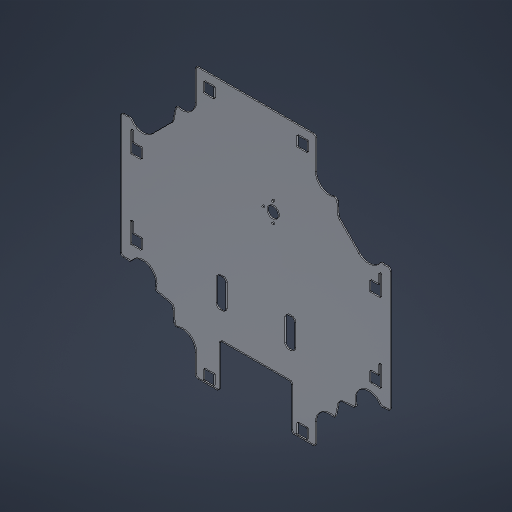
# Autodesk Inventor part: PLATE,BELLYPAN
Saved by Autodesk Inventor 2026 (Build 300175000, 175)
## iProperties
Created: 2026-01-19
Part Number: PLATE,BELLYPAN
Material: Polycarbonate, Clear
Document SubType Name: Sheet Metal
Designer: Jthib
Mass: 1216.4 g
Surface Area: 6786.66 cm^2
Volume: 1013.67 cm^3
Density: 1.2 g/cm^3
Sheet Metal Rule: Default
Appearance: Polycarbonate - Clear
Author: Jthib
Autodesk Inventor part; units mm, degrees
ref_plane "YZ Plane" through (0, 0, 0) normal (1, 0, 0) x (0, 1, 0)
ref_plane "XZ Plane" through (0, 0, 0) normal (0, 1, 0) x (-1, 0, 0)
ref_plane "XY Plane" through (0, 0, 0) normal (0, 0, 1) x (1, 0, 0)
sketch "Sketch1" plane through (0, 0, 0) normal (0, 0, 1) x (1, 0, 0)
  line L0 (-298.45, -349.25) -> (298.45, -349.25)
  line L1 (349.25, -298.45) -> (349.25, 298.45)
  line L2 (298.45, 349.25) -> (-298.45, 349.25)
  line L3 (-349.25, 298.45) -> (-349.25, -298.45)
  line L4 (-349.25, -349.25) -> (349.25, 349.25) construction
  line L5 (349.25, -349.25) -> (-349.25, 349.25) construction
  arc A0 (349.25, 298.45) -> (298.45, 349.25) centre (298.45, 298.45) ccw
  arc A1 (-298.45, 349.25) -> (-349.25, 298.45) centre (-298.45, 298.45) ccw
  arc A2 (-349.25, -298.45) -> (-298.45, -349.25) centre (-298.45, -298.45) ccw
  arc A3 (298.45, -349.25) -> (349.25, -298.45) centre (298.45, -298.45) ccw
  point P0 (0, 0)
  dimension "d0" = 698.5
  dimension "d4" = 50.8
  measures "d0" distance of L4.end L5.end
  measures "d4" radius of A0
extrude "Plate1" add sketch "Sketch1" along normal blind 3.048
sketch "Sketch2" plane through (0, 0, 0) normal (0, 0, -1) x (-1, 0, 0)
  line L0 (-188.9125, -349.25) -> (-336.55, -349.25)
  line L1 (-179.3875, -333.375) -> (-179.3875, -339.725) construction
  arc A0 (-179.3875, -333.375) -> (-188.9125, -323.85) centre (-188.9125, -333.375) ccw construction
  line L2 (-190.5, -323.85) -> (-188.9125, -323.85) construction
  arc A1 (-221.4273, -289.3223) -> (-190.5, -323.85) centre (-190.5, -292.735) ccw construction
  arc A2 (-349.25, -336.55) -> (-336.55, -349.25) centre (-336.55, -336.55) ccw
  line L3 (-349.25, -336.55) -> (-349.25, -188.9125)
  line L4 (-339.725, -179.3875) -> (-333.375, -179.3875) construction
  arc A3 (-323.85, -188.9125) -> (-333.375, -179.3875) centre (-333.375, -188.9125) ccw construction
  line L5 (-323.85, -188.9125) -> (-323.85, -190.5) construction
  arc A4 (-323.85, -190.5) -> (-289.3223, -221.4273) centre (-292.735, -190.5) ccw construction
  arc A5 (-213.9609, -272.2965) -> (-221.4273, -289.3223) centre (-190.5, -292.735) ccw construction
  arc A6 (-213.9609, -272.2965) -> (-211.7954, -264.058) centre (-221.2002, -265.9898) ccw construction
  line L6 (-220.0695, -223.7764) -> (-211.7954, -264.058) construction
  arc A7 (-220.0695, -223.7764) -> (-224.3016, -219.9918) centre (-224.7346, -224.7346) ccw construction
  line L7 (-270.7455, -215.751) -> (-224.3016, -219.9918) construction
  arc A8 (-270.7455, -215.751) -> (-276.598, -217.1034) centre (-271.6186, -225.3124) ccw construction
  arc A9 (-289.3223, -221.4273) -> (-276.598, -217.1034) centre (-292.735, -190.5) ccw construction
  line L8 (-179.3875, -339.725) -> (-179.3875, -349.25) construction
  line L9 (-173.0375, -349.25) -> (-188.9125, -349.25)
  line L10 (-349.25, -188.9125) -> (-349.25, -173.0375)
  line L11 (-349.25, -179.3875) -> (-339.725, -179.3875) construction
  line L12 (-333.375, -173.0375) -> (-339.9898, -173.0375)
  line L13 (-339.9898, -173.0375) -> (-349.25, -173.0375)
  line L14 (-173.0375, -349.25) -> (-173.0375, -339.725)
  line L15 (-173.0375, -339.725) -> (-173.0375, -333.375)
  arc A10 (-173.0375, -333.375) -> (-188.9125, -317.5) centre (-188.9125, -333.375) ccw
  line L16 (-188.9125, -317.5) -> (-190.5, -317.5)
  arc A11 (-215.1156, -290.0188) -> (-190.5, -317.5) centre (-190.5, -292.735) ccw
  arc A12 (-209.1729, -276.4676) -> (-215.1156, -290.0188) centre (-190.5, -292.735) ccw
  arc A13 (-209.1729, -276.4676) -> (-205.5752, -262.7803) centre (-221.2002, -265.9898) ccw
  line L17 (-205.5752, -262.7803) -> (-213.8494, -222.4987)
  arc A14 (-213.8494, -222.4987) -> (-223.7241, -213.6682) centre (-224.7346, -224.7346) ccw
  line L18 (-223.7241, -213.6682) -> (-270.1681, -209.4273)
  arc A15 (-270.1681, -209.4273) -> (-279.8913, -211.6741) centre (-271.6186, -225.3124) ccw
  arc A16 (-290.0188, -215.1156) -> (-279.8913, -211.6741) centre (-292.735, -190.5) ccw
  arc A17 (-317.5, -190.5) -> (-290.0188, -215.1156) centre (-292.735, -190.5) ccw
  line L19 (-317.5, -190.5) -> (-317.5, -188.9125)
  arc A18 (-317.5, -188.9125) -> (-333.375, -173.0375) centre (-333.375, -188.9125) ccw
  line L20 (298.45, -349.25) -> (-298.45, -349.25) construction
  circle A19 centre (-190.5, -292.735) radius 34.925
  circle A20 centre (-292.735, -190.5) radius 34.925
  point P0 (0, 0)
  point P1 (-263.7686, -210.0117)
  point P2 (-324.4183, -175.8055)
  point P3 (-175.8055, -324.4183)
  point P4 (-205.8647, -261.3713)
  dimension "d9" = 6.35
  dimension "d19" = 69.85
  constraints: 40 end point, 38 point on circle, 21 centre point, 5 vertical, 3 horizontal, 3 perpendicular, 2 coincident, 2 collinear, 2 point on line, 1 equal radius, 1 tangent, 55 other
  measures "d9" distance between parallel lines of L17 L6
  measures "d19" diameter of A19
extrude "Cut1" cut sketch "Sketch2" against normal blind 3.048
fillet "Corner Round2" radius 6.35 4 edges at (205.8647, -261.3713, 1.524) (175.8055, -324.4183, 1.524) (263.7686, -210.0117, 1.524) (324.4183, -175.8055, 1.524)
pattern_circular "Circular Pattern1" count 4 over 360 about axis through (0, 0, -10) along (0, 0, 1) of "Cut1", "Corner Round2"
sketch "Sketch3" plane through (0, 0, 0) normal (0, 0, -1) x (-1, 0, 0)
  line L0 (-173.0375, 349.25) -> (173.0375, 349.25) projected
  line L1 (-349.25, -173.0375) -> (-349.25, 173.0375) projected
  point P0 (0, 0)
  point P1 (-44.45, 120.65)
  point P2 (-166.6875, 349.25)
  point P3 (166.6875, 349.25)
  point P4 (-349.25, -166.6875)
  point P5 (-349.25, 166.6875)
  dimension "d10" = 228.6
  dimension "d11" = 304.8
  measures "d10" distance from line of L0 point (-44.45, 120.65)
  measures "d11" distance from line of L1 point (-44.45, 120.65)
hole "Hole1" at (44.45, 120.65, 0) direction (0, 0, 1) diameter 28.575 end through all
sketch "Sketch4" plane through (0, 0, 0) normal (0, 0, -1) x (-1, 0, 0)
  line L0 (173.0375, -349.25) -> (-173.0375, -349.25) construction
  line L1 (93.6625, -349.25) -> (-93.6625, -349.25)
  line L2 (-93.6625, -349.25) -> (-93.6625, -234.95)
  line L3 (-93.6625, -234.95) -> (93.6625, -234.95)
  line L4 (93.6625, -234.95) -> (93.6625, -349.25)
  line L5 (0, -488.95) -> (0, 488.95) construction
  point P0 (0, 0)
  point P1 (166.6875, -349.25)
  point P2 (-166.6875, -349.25)
  dimension "d21" = 187.325
  dimension "d22" = 114.3
  constraints: 8 end point, 2 parallel, 1 horizontal, 1 perpendicular, 1 point on line, 1 other
  measures "d21" distance of L1.start L1.end
  measures "d22" distance of L1.end L2.end
extrude "Cut2" cut sketch "Sketch4" against normal blind 3.048
sketch "Sketch5" plane through (0, 0, 0) normal (0, 0, -1) x (-1, 0, 0)
  line L0 (0, -488.95) -> (0, 488.95) construction
  circle A0 centre (-44.3766, 95.1768) radius 2.0193 construction
  circle A1 centre (-19.05, 120.65) radius 2.0193 construction
  circle A2 centre (-44.5232, 145.9766) radius 2.0193 construction
  point P0 (0, 0)
  constraints: 3 centre point, 6 other
hole "Hole2" at (44.3766, 95.1768, 0) at (19.05, 120.65, 0) at (44.5232, 145.9766, 0) direction (0, 0, 1) diameter 5.1054 end through all start extended yes clearance for "Flat Head Machine Screw (82)" size "#10" standard "Ansi Unified Screw Threads"
sketch "Sketch6" plane through (0, 0, 0) normal (0, 0, -1) x (-1, 0, 0)
  circle A0 centre (-44.5232, 145.9766) radius 2.5527 construction
  circle A1 centre (-19.05, 120.65) radius 2.5527 construction
  circle A2 centre (-44.3766, 95.1768) radius 2.5527 construction
  line L0 (93.6625, -234.95) -> (93.6625, -349.25) construction
  line L1 (173.0375, -349.25) -> (93.6625, -349.25) projected
  line L2 (173.0375, -349.25) -> (173.0375, -333.375) projected
  arc A3 (173.6888, -328.8745) -> (173.0375, -333.375) centre (188.9125, -333.375) ccw projected
  arc A4 (173.6888, -328.8745) -> (171.1225, -321.7913) centre (167.5993, -327.0743) ccw projected
  arc A5 (202.3754, -259.891) -> (171.1225, -321.7913) centre (190.5, -292.735) ccw projected
  arc A6 (202.3754, -259.891) -> (210.8583, -254.4968) centre (204.5346, -253.9193) ccw construction
  line L3 (210.8583, -254.4968) -> (213.6682, -223.7241) construction
  arc A7 (222.4987, -213.8494) -> (213.6682, -223.7241) centre (224.7346, -224.7346) ccw construction
  line L4 (222.4987, -213.8494) -> (254.1305, -207.352) construction
  arc A8 (254.1305, -207.352) -> (258.9885, -199.4962) centre (252.8528, -201.1318) ccw construction
  arc A9 (321.7913, -171.1225) -> (258.9885, -199.4962) centre (292.735, -190.5) ccw construction
  arc A10 (321.7913, -171.1225) -> (328.8745, -173.6888) centre (327.0743, -167.5993) ccw construction
  arc A11 (333.375, -173.0375) -> (328.8745, -173.6888) centre (333.375, -188.9125) ccw construction
  line L5 (333.375, -173.0375) -> (349.25, -173.0375) construction
  line L6 (349.25, 173.0375) -> (349.25, -173.0375) construction
  line L7 (349.25, 173.0375) -> (333.375, 173.0375) construction
  arc A12 (328.8745, 173.6888) -> (333.375, 173.0375) centre (333.375, 188.9125) ccw construction
  arc A13 (328.8745, 173.6888) -> (321.7913, 171.1225) centre (327.0743, 167.5993) ccw construction
  arc A14 (259.891, 202.3754) -> (321.7913, 171.1225) centre (292.735, 190.5) ccw projected
  arc A15 (259.891, 202.3754) -> (254.4968, 210.8583) centre (253.9193, 204.5346) ccw projected
  line L8 (254.4968, 210.8583) -> (223.7241, 213.6682) projected
  arc A16 (213.8494, 222.4987) -> (223.7241, 213.6682) centre (224.7346, 224.7346) ccw projected
  line L9 (213.8494, 222.4987) -> (207.352, 254.1305) construction
  arc A17 (207.352, 254.1305) -> (199.4962, 258.9885) centre (201.1318, 252.8528) ccw construction
  arc A18 (171.1225, 321.7913) -> (199.4962, 258.9885) centre (190.5, 292.735) ccw projected
  arc A19 (171.1225, 321.7913) -> (173.6888, 328.8745) centre (167.5993, 327.0743) ccw projected
  arc A20 (173.0375, 333.375) -> (173.6888, 328.8745) centre (188.9125, 333.375) ccw projected
  line L10 (173.0375, 333.375) -> (173.0375, 349.25) projected
  line L11 (-173.0375, 349.25) -> (173.0375, 349.25) projected
  line L12 (-173.0375, 349.25) -> (-173.0375, 333.375) projected
  arc A21 (-173.6888, 328.8745) -> (-173.0375, 333.375) centre (-188.9125, 333.375) ccw projected
  arc A22 (-173.6888, 328.8745) -> (-171.1225, 321.7913) centre (-167.5993, 327.0743) ccw projected
  arc A23 (-202.3754, 259.891) -> (-171.1225, 321.7913) centre (-190.5, 292.735) ccw projected
  arc A24 (-202.3754, 259.891) -> (-210.8583, 254.4968) centre (-204.5346, 253.9193) ccw construction
  line L13 (-210.8583, 254.4968) -> (-213.6682, 223.7241) construction
  arc A25 (-222.4987, 213.8494) -> (-213.6682, 223.7241) centre (-224.7346, 224.7346) ccw projected
  line L14 (-222.4987, 213.8494) -> (-254.1305, 207.352) projected
  arc A26 (-254.1305, 207.352) -> (-258.9885, 199.4962) centre (-252.8528, 201.1318) ccw projected
  arc A27 (-321.7913, 171.1225) -> (-258.9885, 199.4962) centre (-292.735, 190.5) ccw projected
  arc A28 (-321.7913, 171.1225) -> (-328.8745, 173.6888) centre (-327.0743, 167.5993) ccw construction
  arc A29 (-333.375, 173.0375) -> (-328.8745, 173.6888) centre (-333.375, 188.9125) ccw construction
  line L15 (-333.375, 173.0375) -> (-349.25, 173.0375) construction
  line L16 (-349.25, -173.0375) -> (-349.25, 173.0375) construction
  line L17 (-349.25, -173.0375) -> (-333.375, -173.0375) construction
  arc A30 (-328.8745, -173.6888) -> (-333.375, -173.0375) centre (-333.375, -188.9125) ccw construction
  arc A31 (-328.8745, -173.6888) -> (-321.7913, -171.1225) centre (-327.0743, -167.5993) ccw construction
  arc A32 (-259.891, -202.3754) -> (-321.7913, -171.1225) centre (-292.735, -190.5) ccw construction
  arc A33 (-259.891, -202.3754) -> (-254.4968, -210.8583) centre (-253.9193, -204.5346) ccw construction
  line L18 (-254.4968, -210.8583) -> (-223.7241, -213.6682) construction
  arc A34 (-213.8494, -222.4987) -> (-223.7241, -213.6682) centre (-224.7346, -224.7346) ccw construction
  line L19 (-213.8494, -222.4987) -> (-207.352, -254.1305) construction
  arc A35 (-207.352, -254.1305) -> (-199.4962, -258.9885) centre (-201.1318, -252.8528) ccw construction
  arc A36 (-171.1225, -321.7913) -> (-199.4962, -258.9885) centre (-190.5, -292.735) ccw projected
  arc A37 (-171.1225, -321.7913) -> (-173.6888, -328.8745) centre (-167.5993, -327.0743) ccw projected
  arc A38 (-173.0375, -333.375) -> (-173.6888, -328.8745) centre (-188.9125, -333.375) ccw projected
  line L20 (-173.0375, -333.375) -> (-173.0375, -349.25) projected
  line L21 (-93.6625, -349.25) -> (-173.0375, -349.25) projected
  line L22 (-93.6625, -349.25) -> (-93.6625, -234.95) construction
  line L23 (-93.6625, -234.95) -> (93.6625, -234.95) construction
  circle A39 centre (-44.45, 120.65) radius 14.2875 construction
  line L24 (155.575, -292.735) -> (155.575, -349.25)
  line L25 (-155.575, -349.25) -> (-155.575, -292.735)
  line L26 (-93.6625, -349.25) -> (-173.0375, -349.25) projected
  line L27 (155.575, 292.735) -> (155.575, 349.25)
  line L28 (-155.575, 292.735) -> (-155.575, 349.25)
  line L29 (268.061, 165.7826) -> (216.8838, 216.87)
  line L30 (-216.8838, 216.87) -> (-268.061, 165.7826)
  point P0 (0, 0)
  constraints: 12 end point, 8 point on circle, 8 tangent, 4 perpendicular, 4 point on line
extrude "Cut3" cut sketch "Sketch6" against normal blind 3.048
move faces "Move1" translate (0, -25.4, 0) faces at (-176.1603, 39.0974, 0) (-233.9429, 199.8409, 1.016) (-216.3906, 217.3953, 2.032) (-209.5178, 243.5865, 2.032) (-158.0862, 279.7312, 2.032) (-155.575, 330.4117, 1.016) (-285.9517, 156.2401, 2.032) (-325.3406, 173.7081, 2.032) (-329.3629, 173.5529, 1.016) (-338.6667, 173.0375, 1.016) (-206.407, 256.3877, 1.016) (251.0019, 182.8117, 1.016) (306.1288, 158.2453, 2.032) (213.7791, 222.8732, 2.032) (212.7315, 233.9817, 1.016) (210.3944, 256.3658, 1.016) (171.4652, 263.4531, 2.032) (155.575, 311.5733, 1.016) (324.4927, 173.4009, 2.032) (330.8507, 173.2395, 2.032) (343.9583, 173.0375, 1.016)
sketch "Sketch7" plane through (155.575, 349.25, 0) normal (0, 0, -1) x (-1, 0, 0)
  line L0 (155.575, -838.2) -> (155.575, 139.7) construction
  line L1 (0, 0) -> (311.15, 0) construction
  line L2 (479.425, -432.1175) -> (479.425, -482.2825)
  line L3 (477.8375, -483.87) -> (453.0725, -483.87)
  line L4 (451.485, -482.2825) -> (451.485, -458.7875)
  line L5 (453.0725, -457.2) -> (473.075, -457.2)
  line L6 (474.6625, -455.6125) -> (474.6625, -432.1175)
  line L7 (476.25, -430.53) -> (477.8375, -430.53)
  line L8 (504.825, -201.6125) -> (504.825, -522.2875) construction
  arc A0 (479.425, -432.1175) -> (477.8375, -430.53) centre (477.8375, -432.1175) ccw
  arc A1 (476.25, -430.53) -> (474.6625, -432.1175) centre (476.25, -432.1175) ccw
  arc A2 (473.075, -457.2) -> (474.6625, -455.6125) centre (473.075, -455.6125) ccw
  arc A3 (453.0725, -457.2) -> (451.485, -458.7875) centre (453.0725, -458.7875) ccw
  arc A4 (451.485, -482.2825) -> (453.0725, -483.87) centre (453.0725, -482.2825) ccw
  arc A5 (477.8375, -483.87) -> (479.425, -482.2825) centre (477.8375, -482.2825) ccw
  arc A6 (273.7282, -685.927) -> (278.7218, -685.927) centre (276.225, -685.8) ccw construction
  line L9 (262.89, -668.02) -> (289.56, -668.02)
  line L10 (289.56, -668.02) -> (289.56, -694.69)
  line L11 (289.56, -694.69) -> (262.89, -694.69)
  line L12 (262.89, -694.69) -> (262.89, -668.02)
  line L13 (262.89, -668.02) -> (289.56, -694.69) construction
  line L14 (289.56, -668.02) -> (262.89, -694.69) construction
  line L15 (311.15, -698.5) -> (249.2375, -698.5) construction
  point P0 (155.575, -349.25)
  point P1 (479.425, -430.53)
  point P2 (479.425, -483.87)
  point P3 (451.485, -483.87)
  point P4 (474.6625, -457.2)
  point P5 (474.6625, -430.53)
  point P6 (276.225, -681.355)
  dimension "d44" = 4.7625
  dimension "d45" = 53.34
  dimension "d46" = 26.67
  dimension "d47" = 25.4
  dimension "d48" = 27.94
  dimension "d49" = 1.5875
  dimension "d55" = 26.67
  dimension "d56" = 26.67
  dimension "d57" = 3.81
  dimension "d64" = 134.62
  constraints: 24 end point, 14 point on circle, 12 tangent, 10 point on line, 7 centre point, 6 perpendicular, 5 equal radius, 2 midpoint, 2 parallel, 1 horizontal, 1 vertical, 1 vertical alignment, 4 other
  measures "d44" distance of point (474.663, -430.53) point (479.425, -430.53)
  measures "d45" distance of point (479.425, -430.53) point (479.425, -483.87)
  measures "d46" distance of point (474.663, -457.2) point (474.663, -430.53)
  measures "d47" distance between parallel lines of L8 L2
  measures "d48" distance of point (479.425, -483.87) point (451.485, -483.87)
  measures "d49" radius of A0
  measures "d55" distance of L10.end L11.end
  measures "d56" distance of L10.end L9.end
  measures "d57" distance between parallel lines of L15 L11
  measures "d64" distance from line of point (155.575, -349.25) L3
extrude "Cut4" cut sketch "Sketch7" against normal blind 3.048 contours L2 A5 L3 A4 L4 A3 L5 A2 L6 A1 L7 A0
pattern_linear "Rectangular Pattern1" count 2 spacing 203.2 along (0, 1, 0) of "Cut4"
extrude "Cut5" cut sketch "Sketch7" against normal blind 3.048 contours L9 L10 L11 L12
pattern_linear "Rectangular Pattern2" count 2 spacing 644.525 along (0, 1, 0) of "Cut5"
sketch "Sketch8" plane through (155.575, 349.25, 0) normal (0, 0, -1) x (-1, 0, 0)
  line L0 (257.175, -514.35) -> (231.775, -514.35)
  line L1 (231.775, -514.35) -> (231.775, -438.15)
  line L2 (231.775, -438.15) -> (257.175, -438.15)
  line L3 (257.175, -438.15) -> (257.175, -514.35)
  line L4 (257.175, -514.35) -> (231.775, -438.15) construction
  line L5 (231.775, -514.35) -> (257.175, -438.15) construction
  line L6 (155.575, -838.2) -> (155.575, 139.7) construction
  line L7 (644.525, -349.25) -> (-333.375, -349.25) construction
  point P0 (155.575, -349.25)
  point P1 (244.475, -476.25)
  dimension "d66" = 76.2
  dimension "d67" = 25.4
  dimension "d68" = 76.2
  dimension "d69" = 127
  constraints: 12 end point, 2 midpoint, 2 parallel, 1 horizontal, 1 perpendicular
  measures "d66" distance of L0.end L1.end
  measures "d67" distance of L0.start L0.end
  measures "d68" distance between parallel lines of L6 L1
  measures "d69" distance from line of L7 point (244.475, -476.25)
extrude "Cut6" cut sketch "Sketch8" against normal blind 3.048
mirror "Mirror1" about plane through (0, 0, 0) normal (1, 0, 0) of "Cut4", "Rectangular Pattern1", "Cut5", "Rectangular Pattern2", "Cut6"
fillet "Corner Round3" radius 6.35 12 edges at (93.6625, -234.95, 1.524) (-93.6625, -234.95, 1.524) (-349.25, -173.0375, 1.524) (-349.25, 147.6375, 1.524) (349.25, -173.0375, 1.524) (349.25, 147.6375, 1.524) (-93.6625, -349.25, 1.524) (93.6625, -349.25, 1.524) (155.575, 349.25, 1.524) (-155.575, 349.25, 1.524) (-155.575, -349.25, 1.524) (155.575, -349.25, 1.524)
fillet "Corner Round4" radius 1.5875 16 edges at (-133.985, -318.77, 1.524) (-107.315, -318.77, 1.524) (-133.985, 299.085, 1.524) (-107.315, 299.085, 1.524) (-133.985, 325.755, 1.524) (-107.315, 325.755, 1.524) (107.315, 299.085, 1.524) (133.985, 299.085, 1.524) (107.315, 325.755, 1.524) (133.985, 325.755, 1.524) (107.315, -318.77, 1.524) (133.985, -318.77, 1.524) (-133.985, -345.44, 1.524) (-107.315, -345.44, 1.524) (107.315, -345.44, 1.524) (133.985, -345.44, 1.524)
fillet "Corner Round5" radius 9.525 8 edges at (-101.6, -165.1, 1.524) (-76.2, -165.1, 1.524) (-101.6, -88.9, 1.524) (-76.2, -88.9, 1.524) (101.6, -165.1, 1.524) (76.2, -165.1, 1.524) (101.6, -88.9, 1.524) (76.2, -88.9, 1.524)
equation "\"d2\" = Thickness"
equation "\"d17\" = Thickness"
equation "\"d23\" = Thickness"
equation "\"d33\" = Thickness"
equation "\"d36\" = Thickness"
equation "\"d46\" = 0.5 * d45"
equation "\"d50\" = Thickness"
equation "\"d59\" = Thickness"
equation "\"d70\" = Thickness"
equation "\"d1\" = Thickness"
equation "\"BendRadius\" = Thickness"
equation "\"BendReliefWidth\" = Thickness"
equation "\"BendReliefDepth\" = 0.5 * Thickness"
equation "\"CornerReliefSize\" = 4 * Thickness"
equation "\"MinimumRemnant\" = 2 * Thickness"
equation "\"TransitionRadius\" = BendRadius"
equation "\"JacobiRadiusSize\" = BendRadius"
equation "\"GapSize\" = Thickness"
equation "\"Thickness\" = 3.048"
body "Solid1"
